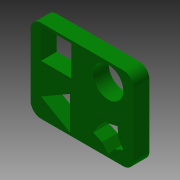
# Autodesk Inventor part: PassemgerBaseDE
Saved by Autodesk Inventor 2015 (Build 190159000, 159)
## iProperties
Created: 2017-12-01
Part Number: PassemgerBaseDE
Material: ABS Plastic
Document SubType Name: Modeling
Designer: Administrator
Density: 1.06 g/cm^3
Appearance: Smooth - Dark Forest Green
Mass: 1.11827 g
Surface Area: 84.0144 cm^2
Volume: 1.05497 cm^3
Author: Administrator
Autodesk Inventor part; units mm, degrees
ref_plane "YZ Plane" through (0, 0, 0) normal (1, 0, 0) x (0, 1, 0)
ref_plane "XZ Plane" through (0, 0, 0) normal (0, 1, 0) x (-1, 0, 0)
ref_plane "XY Plane" through (0, 0, 0) normal (0, 0, 1) x (1, 0, 0)
sketch "Sketch1" plane through (0, 0, 0) normal (0, 0, 1) x (1, 0, 0)
  line L0 (5.08, 0) -> (45.085, 0)
  line L1 (50.165, 5.08) -> (50.165, 35.306)
  line L2 (45.085, 40.386) -> (5.08, 40.386)
  line L3 (0, 35.306) -> (0, 5.08)
  arc A0 (5.08, 40.386) -> (0, 35.306) centre (5.08, 35.306) ccw
  arc A1 (50.165, 35.306) -> (45.085, 40.386) centre (45.085, 35.306) ccw
  arc A2 (45.085, 0) -> (50.165, 5.08) centre (45.085, 5.08) ccw
  arc A3 (0, 5.08) -> (5.08, 0) centre (5.08, 5.08) ccw
  circle A4 centre (12.446, 31.75) radius 7.366
  line L4 (30.353, 39.116) -> (45.085, 39.116)
  line L5 (45.085, 39.116) -> (45.085, 24.384)
  line L6 (45.085, 24.384) -> (30.353, 24.384)
  line L7 (30.353, 24.384) -> (30.353, 39.116)
  line L8 (31.0509, 17.4752) -> (31.0509, 1.27)
  line L9 (31.0509, 1.27) -> (45.085, 9.3726)
  line L10 (45.085, 9.3726) -> (31.0509, 17.4752)
  circle A5 centre (12.3952, 9.2202) radius 5.2324 construction
  circle A6 centre (12.3952, 9.2202) radius 7.6835 construction
  line L11 (12.3952, 1.5367) -> (15.4707, 4.9871)
  line L12 (15.4707, 4.9871) -> (19.7026, 6.8459)
  line L13 (19.7026, 6.8459) -> (17.3715, 10.8371)
  line L14 (17.3715, 10.8371) -> (16.9114, 15.4363)
  line L15 (16.9114, 15.4363) -> (12.3952, 14.4526)
  line L16 (7.879, 15.4363) -> (7.4189, 10.8371)
  line L17 (7.4189, 10.8371) -> (5.0878, 6.8459)
  line L18 (5.0878, 6.8459) -> (9.3197, 4.9871)
  line L19 (9.3197, 4.9871) -> (12.3952, 1.5367)
  line L20 (7.879, 15.4363) -> (12.3952, 14.4526)
  point P0 (0, 0)
  point P1 (50.165, 0)
  point P2 (0, 40.386)
  dimension "d17" = 10.4648
  dimension "d18" = 15.367
  dimension "d0" = 40.386
  dimension "d1" = 50.165
  dimension "d2" = 5.08
  dimension "d3" = 14.732
  dimension "d4" = 8.636
  dimension "d5" = 12.446
  dimension "d6" = 14.732
  dimension "d7" = 14.732
  dimension "d8" = 1.27
  dimension "d9" = 5.08
  dimension "d10" = 16.2052
  dimension "d12" = 5.08
  dimension "d13" = 1.27
  dimension "d15" = 16.2052
  dimension "d16" = 16.2052
  dimension "d21" = 360
  dimension "d25" = 360
  dimension "d27" = 9.2202
  dimension "d28" = 12.3952
  constraints: 42 end point, 8 point on circle, 8 tangent, 6 point on line, 5 centre point, 4 parallel, 3 equal radius, 2 horizontal, 2 perpendicular, 2 vertical alignment, 1 coincident, 1 vertical, 16 other
  measures "d0" distance of point (0, 40.386) point (0, 0)
  measures "d1" distance of point (0, 0) point (50.165, 0)
  measures "d2" radius of A0
  measures "d3" diameter of A4
  measures "d4" distance from line of L2 A4.centre
  measures "d5" distance from line of A4.centre L3
  measures "d6" distance of L5.end L6.end
  measures "d7" distance of L6.end L4.start
  measures "d8" distance between parallel lines of L4 L2
  measures "d9" distance between parallel lines of L1 L5
  measures "d10" distance of L8.start L8.end
  measures "d12" distance from line of L1 L9.end
  measures "d13" distance from line of L0 L8.end
  measures "d15" distance of L9.end L8.start
  measures "d16" distance of L9.end L8.end
  measures "d27" distance from line of L0 point (12.395, 9.22)
  measures "d28" distance from line of L3 point (12.395, 9.22)
extrude "Extrusion1" add sketch "Sketch1" along normal blind 7.62
shell "Shell1" thickness 0.254 removed faces 1 at (40.407, 17.0773, 7.62)
body "Solid1"
